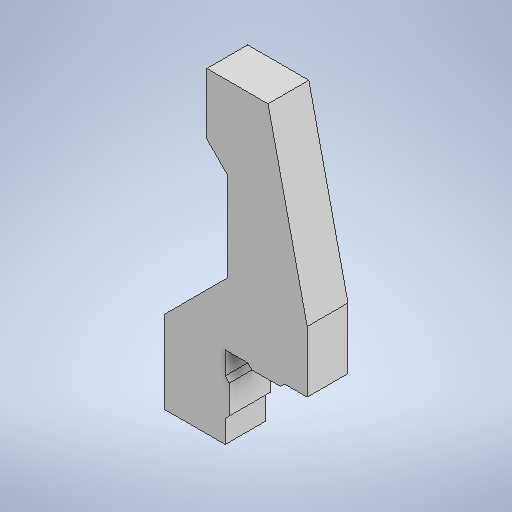
# Autodesk Inventor part: Z-Endstop
Saved by Autodesk Inventor 2025.3 (Build 293356030, 356C)
## iProperties
Created: 2025-10-01
Part Number: Z-Endstop
Material: Generic
Document SubType Name: Modeling
Designer: tvoko
Density: 1 g/cm^3
Appearance: Default
Author: tvoko
Autodesk Inventor part; units mm, degrees
ref_plane "YZ Plane" through (0, 0, 0) normal (1, 0, 0) x (0, 1, 0)
ref_plane "XZ Plane" through (0, 0, 0) normal (0, 1, 0) x (-1, 0, 0)
ref_plane "XY Plane" through (0, 0, 0) normal (0, 0, 1) x (1, 0, 0)
sketch "Sketch1" plane through (0, 0, 0) normal (0, 0, 1) x (1, 0, 0)
  line L0 (-10.05, 10.05) -> (10.05, 10.05)
  line L1 (10.05, 10.05) -> (10.05, -10.05)
  line L2 (10.05, -10.05) -> (-10.05, -10.05)
  line L3 (-10.05, -10.05) -> (-10.05, 10.05)
  line L4 (0, 10.05) -> (0, -10.05) construction
  line L5 (-10.05, 0) -> (10.05, 0) construction
  line L6 (-10.05, 4.5) -> (-9.05, 3.5)
  line L7 (-9.05, 3.5) -> (-9.05, -3.5)
  line L8 (-9.05, -3.5) -> (-10.05, -4.5)
  line L9 (-4.5, 10.05) -> (-3.5, 9.05)
  line L10 (-3.5, 9.05) -> (3.5, 9.05)
  line L11 (3.5, 9.05) -> (4.5, 10.05)
  line L12 (10.05, 10.05) -> (10.05, 25.05)
  line L13 (-10.05, -10.05) -> (-25.05, -10.05)
  line L14 (-14.55, 52.55) -> (-14.55, 67.55)
  line L15 (-14.55, 67.55) -> (0.45, 67.55)
  line L16 (0.45, 67.55) -> (10.05, 25.05)
  line L17 (-14.55, 60.05) -> (-7.05, 60.05) construction
  line L18 (-7.05, 60.05) -> (-7.05, 67.55) construction
  line L19 (-25.05, -10.05) -> (-25.05, 10.05)
  line L20 (-14.55, 52.55) -> (-9.55, 47.55)
  line L21 (-9.55, 47.55) -> (-9.55, 25.55)
  line L22 (-9.55, 25.55) -> (-25.05, 10.05)
  point P0 (0, 0)
  point P1 (0, 0)
  point P2 (0, 9.05)
  point P3 (-9.05, 0)
  dimension "d0" = 20.1
  dimension "d1" = 7
  dimension "d2" = 1
  dimension "d3" = 135
  dimension "d4" = 1
  dimension "d5" = 7
  dimension "d6" = 135
  dimension "d7" = 15
  dimension "d8" = 15
  dimension "d9" = 15
  dimension "d11" = 50
  dimension "d14" = 135
  dimension "d16" = 5
  dimension "d17" = 3
  constraints: 46 end point, 9 midpoint, 6 perpendicular, 6 point on line, 5 equal length, 4 horizontal, 3 vertical, 2 parallel, 1 coincident
  measures "d0" distance of L0.start L0.end
  measures "d1" distance of L9.end L10.end
  measures "d2" distance between parallel lines of L0 L10
  measures "d3" angle of L10 L11
  measures "d4" distance between parallel lines of L3 L7
  measures "d5" distance of L6.end L7.end
  measures "d6" angle of L7 L6
  measures "d7" distance of L14.end L15.end
  measures "d8" distance of L2.end L13.end
  measures "d9" distance of L0.end L12.end
  measures "d11" distance between parallel lines of L0 L17
  measures "d14" angle of L20 L21
  measures "d16" distance between parallel lines of L14 L21
  measures "d17" distance between parallel lines of L3 L18
extrude "Extrusion1" add sketch "Sketch1" along normal blind 10 contours L3 L13 L19 L22 L21 L20 L14 L15 L16 L12 L0 | L0 L11 L10 L9 | L6 L7 L8 L3
body "Solid1"
